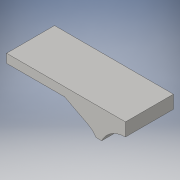
# Autodesk Inventor part: Antibuckler
Saved by Autodesk Inventor 2016 (Build 200138000, 138)
## iProperties
Created: 2016-04-02
Part Number: Antibuckler
Material: Generic
Document SubType Name: Modeling
Designer: Scott
Density: 1 g/cm^3
Appearance: Default
Author: Scott
Autodesk Inventor part; units mm, degrees
ref_plane "YZ Plane" through (0, 0, 0) normal (1, 0, 0) x (0, 1, 0)
ref_plane "XZ Plane" through (0, 0, 0) normal (0, 1, 0) x (-1, 0, 0)
ref_plane "XY Plane" through (0, 0, 0) normal (0, 0, 1) x (1, 0, 0)
sketch "Sketch1" plane through (0, 0, 0) normal (0, 0, 1) x (1, 0, 0)
  arc A0 (5.1036, 3.2163) -> (2.772, 5.3579) centre (0, 0) ccw
  arc A1 (13.6525, 7.62) -> (6.7446, 3.2163) centre (13.6525, 0) ccw
  line L0 (13.6525, 11.43) -> (0, 11.43)
  line L1 (-20.955, 11.43) -> (0, 11.43)
  line L2 (5.1036, 3.2163) -> (6.7446, 3.2163)
  line L3 (-20.955, 11.43) -> (-20.955, 8.89)
  line L4 (-20.955, 8.89) -> (-4.055, 8.89)
  line L5 (-4.055, 8.89) -> (2.772, 5.3579)
  line L6 (13.6525, 7.62) -> (13.6525, 11.43)
  dimension "d0" = 12.065
  dimension "d4" = 2.54
  constraints: 14 end point, 4 point on circle, 2 centre point, 2 tangent, 1 coincident, 1 horizontal, 1 perpendicular, 1 vertical
  measures "d0" diameter of A0
  measures "d4" distance of L1.start L3.end
extrude "Extrusion1" add sketch "Sketch1" along normal blind 13.97
sketch "Sketch2" plane through (5.1036, 3.2163, 0) normal (0, -1, 0) x (1, 0, 0)
  point P0 (-5.1036, 0)
body "Solid1"
